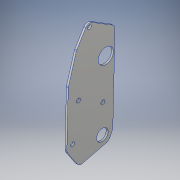
# Autodesk Inventor part: Module Plate 1
Saved by Autodesk Inventor 2019.4 (Build 234330000, 330)
## iProperties
Created: 2019-10-19
Part Number: Module Plate 1
Material: Aluminum 6061
Document SubType Name: Modeling
Designer: admin
Density: 2.7 g/cm^3
Appearance: Aluminum - Flat
Mass: 225.839 g
Surface Area: 449.408 cm^2
Volume: 83.6441 cm^3
Height: 75.000 mm
Author: admin
Autodesk Inventor part; units mm, degrees
ref_plane "YZ Plane" through (0, 0, 0) normal (1, 0, 0) x (0, 1, 0)
ref_plane "XZ Plane" through (0, 0, 0) normal (0, 1, 0) x (-1, 0, 0)
ref_plane "XY Plane" through (0, 0, 0) normal (0, 0, 1) x (1, 0, 0)
sketch "Sketch1" plane through (0, 0, 0) normal (1, 0, 0) x (0, 1, 0)
  circle A0 centre (0, 0) radius 62.5 construction
  circle A1 centre (-143.0555, 7.5) radius 50 construction
  line L0 (-143.0555, 7.5) -> (0, 0) construction
  line L1 (-161.7434, -42.5) -> (-102.4467, -42.5) construction
  line L2 (-16.0459, -62.5) -> (40.9165, -62.5) construction
  line L3 (-160.8345, -6.0612) -> (-142.874, -14.8599)
  line L4 (-142.874, -14.8599) -> (-73.1769, -16.662)
  line L5 (46.5314, -19.7571) -> (81.8069, 37.8501)
  line L6 (81.8069, 37.8501) -> (13.4998, 79.6777)
  line L7 (13.4998, 79.6777) -> (-137.4135, 83.5796)
  line L8 (-137.4135, 83.5796) -> (-176.516, 57.3036)
  line L9 (-176.516, 57.3036) -> (-160.8345, -6.0612)
  circle A2 centre (0, 0) radius 16.3
  circle A3 centre (-143.0555, 7.5) radius 12.3
  line L10 (-151.8542, -10.4606) -> (-143.0555, 7.5) construction
  arc A4 (-61.867, -16.9544) -> (-73.1769, -16.662) centre (-67.341, -9.8105) ccw construction
  line L11 (-98.4698, -16.008) -> (-97.8311, -16.0245) construction
  line L12 (-97.8311, -16.0245) -> (-61.867, -16.9544) construction
  line L13 (-61.867, -16.9544) -> (-98.4698, -16.008) construction
  line L14 (-73.1769, -16.662) -> (46.5314, -19.7571)
  line L15 (0, 0) -> (-212.6616, 0) construction
  circle A5 centre (-83.0555, 6.6011) radius 4.25
  dimension "d0" = 125
  dimension "d1" = 100
  dimension "d2" = 143.252
  dimension "d3" = 20
  dimension "d4" = 20
  dimension "d5" = 32.6
  dimension "d6" = 24.6
  dimension "d7" = 23.099
  dimension "d8" = 20
  dimension "d9" = 130
  dimension "d10" = 110
  dimension "d12" = 155.381
  dimension "d13" = 80
  dimension "d14" = 90
  dimension "d15" = 150
  dimension "Height" = 75
  dimension "d17" = 50
  dimension "d18" = 60
  dimension "d30" = 8.5
  dimension "d31" = 23
  dimension "d32" = 60
  constraints: 32 end point, 6 centre point, 5 parallel, 4 point on line, 3 coincident, 3 horizontal, 2 point on circle, 2 tangent, 1 midpoint, 1 perpendicular
  measures "d0" diameter of A0
  measures "d1" diameter of A1
  measures "d2" distance of L0.start L0.end
  measures "d3" distance between parallel lines of L2 L1
  measures "d4" distance from line of L0.start L3
  measures "d5" diameter of A2
  measures "d6" diameter of A3
  measures "d7" angle of L0 L3
  measures "d8" distance of L3.start L3.end
  measures "d9" angle of L3 L9
  measures "d10" angle of L9 L8
  measures "d12" angle of L4 L3
  measures "d13" distance from line of L15.start L7
  measures "d14" angle of L5 L6
  measures "d15" angle of L7 L6
  measures "Height" distance from line of point (0, 0) L6
  measures "d17" distance from line of L15.start L5
  measures "d18" distance from line of L10.end L8
  measures "d30" diameter of A5
  measures "d31" distance from line of L4 A5.centre
  measures "d32" horizontal distance of L0.start A5.centre
extrude "Extrusion1" add sketch "Sketch1" along normal blind 4
fillet "Fillet3" radius 10 6 edges at (2, 81.8069, 37.8501) (2, 46.5314, -19.7571) (2, -142.874, -14.8599) (2, -160.8345, -6.0612) (2, -176.516, 57.3036) (2, -137.4135, 83.5796)
chamfer "Chamfer1" distance 32 angle 45 1 edges at (2, 13.4998, 79.6777)
fillet "Fillet4" radius 10 2 edges at (2, 40.7898, 62.9668) (2, -18.4895, 80.5048)
sketch "Sketch2" plane through (4, 0, 0) normal (1, 0, 0) x (0, 0, -1)
  circle A0 centre (0, 0) radius 16.3
  circle A1 centre (0, 0) radius 16.3 projected
  circle A2 centre (-71.4855, -128.5174) radius 4.25
  line L0 (-81.8006, -140.0609) -> (-61.209, -170.7042) projected
  line L1 (-50.5066, -174.8339) -> (1.5347, -161.9548) projected
  circle A3 centre (-35.2054, 70.8067) radius 4.25
  arc A4 (-29.322, 76.5847) -> (-43.0723, 73.2788) centre (-34.5442, 68.0566) ccw projected
  line L2 (14.8333, 49.5464) -> (-29.322, 76.5847) projected
  line L3 (-43.0723, 73.2788) -> (-62.2792, 41.9126) projected
  circle A5 centre (-58.9603, -53.5174) radius 4.25
  line L4 (-58.9603, -53.5174) -> (-71.4855, -128.5174)
  line L5 (-80.5388, -19.8056) -> (-83.4971, -134.225) projected
  point P0 (18.0192, 10.7846)
  point P1 (18.8908, -9.1727)
  dimension "d39" = 32.6
  dimension "d42" = 8.5
  dimension "d43" = 15
  dimension "d44" = 50
  dimension "d45" = 8.5
  dimension "d47" = 8
  dimension "d48" = 8
  dimension "d49" = 8.5
  dimension "d50" = 8
  dimension "d51" = 75
  constraints: 4 centre point, 2 end point, 2 other
  measures "d39" diameter of A0
  measures "d42" diameter of A2
  measures "d43" distance from line of L0 L4.end
  measures "d44" distance from line of L1 L4.end
  measures "d45" diameter of A3
  measures "d47" distance from line of L2 A3.centre
  measures "d48" distance from line of L3 A3.centre
  measures "d49" diameter of A5
  measures "d50" angle of L5 L4
  measures "d51" vertical distance of L4.end L4.start
extrude "Extrusion2" cut sketch "Sketch2" against normal blind 9.5
body "Solid1"
